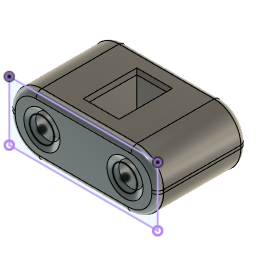
Schiebemechanismus Regler (Autodesk Fusion 360 design; units mm, degrees)
Autodesk Fusion 360 part; units mm, degrees
box "Grundkörper Quader1" add length 30 width 50 height 20 placed x (0, 1, 0) y (-1, 0, 0) z (0, 0, 1) at (50, 0, 0)
sketch "Skizze2" plane through (0, 0, 0) normal (0, -1, 0) x (1, 0, 0)
  line L0 (0, 20) -> (0, 0)
  line L1 (0, 0) -> (50, 0)
  line L2 (50, 0) -> (50, 20)
  line L3 (50, 20) -> (0, 20)
sketch "Skizze3" plane through (0, 0, 0) normal (0, -1, 0) x (1, 0, 0)
  circle A0 centre (11, 10) radius 4.1
  circle A1 centre (39, 10) radius 4.1
  line L0 (0, 20) -> (0, 0)
  line L1 (50, 0) -> (50, 20)
  line L2 (50, 20) -> (0, 20)
  line L3 (50, 0) -> (0, 0)
  dimension "d6" = 8.2
  dimension "d7" = 8.2
  dimension "d8" = 28
  dimension "d10" = 11
  dimension "d11" = 10
  dimension "d23" = 10
  measures "d6" diameter of A0
  measures "d7" diameter of A1
  measures "d8" distance of A0.centre A1.centre
  measures "d10" distance of A1.centre L1
  measures "d11" distance of A0.centre L2
  measures "d23" distance of A1.centre L3
hole "Bohrung1" at (11, 0, 10) direction (0, 1, 0) diameter 8.2 depth 30 tip angle 118
sketch "Skizze4" plane through (0, 0, 0) normal (0, -1, 0) x (1, 0, 0)
hole "Bohrung2" at (39, 0, 10) direction (0, 1, 0) diameter 8.2 depth 30 tip angle 118
fillet "Abrundung1" radius 9 2 edges at (0, 15, 20) (50, 15, 20)
fillet "Abrundung2" radius 10 2 edges at (50, 15, 0) (0, 15, 0)
fillet "Abrundung3" radius 2 8 edges at (50, 0, 10.5) (47.0711, 0, 2.9289) (25, 0, 0) (2.9289, 0, 2.9289) (0, 0, 10.5) (2.636, 0, 17.364) (25, 0, 20) (47.364, 0, 17.364)
fillet "Abrundung4" radius 2 8 edges at (0, 30, 10.5) (2.9289, 30, 2.9289) (25, 30, 0) (47.0711, 30, 2.9289) (50, 30, 10.5) (47.364, 30, 17.364) (25, 30, 20) (2.636, 30, 17.364)
chamfer "Fase1" distance 2 angle 45 2 edges at (37.5174, 30, 13.8225) (9.5174, 30, 13.8225)
chamfer "Fase2" distance 2 angle 45 2 edges at (12.4826, 0, 13.8225) (40.4826, 0, 13.8225)
sketch "Skizze5" plane through (0, 0, 20) normal (0, 0, 1) x (-1, 0, 0)
  line L0 (-41, -28) -> (-9, -28)
  line L1 (-9, -28) -> (-9, -2)
  line L2 (-9, -2) -> (-41, -2)
  line L3 (-41, -2) -> (-41, -28)
  line L4 (-29.951, -7) -> (-29.951, -23)
  line L5 (-29.951, -23) -> (-19.951, -23)
  line L6 (-19.951, -23) -> (-19.951, -7)
  line L7 (-19.951, -7) -> (-29.951, -7)
  constraint vertical L4
  constraint perpendicular L4 L5
  constraint perpendicular L5 L6
  constraint perpendicular L4 L7
extrude "Extrusion1" cut sketch "Skizze5" against normal blind 32 contours L4 L5 L6 L7
chamfer "Fase3" distance 1 angle 45 4 edges at (19.951, 15, 20) (29.951, 15, 20) (24.951, 7, 20) (24.951, 23, 20)
